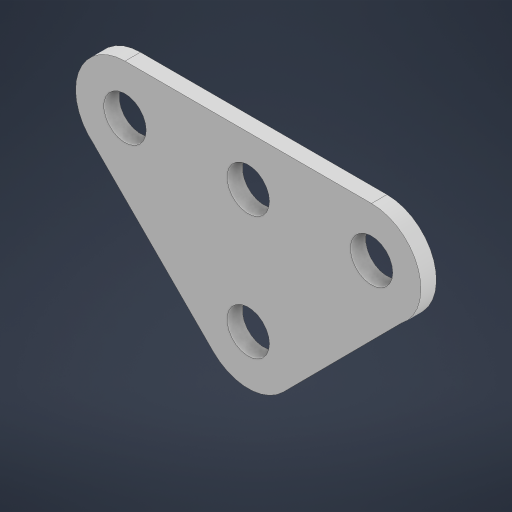
# Autodesk Inventor part: Wing poly connection
Saved by Autodesk Inventor 2023.4 (Build 274418000, 418)
## iProperties
Created: 2024-01-13
Part Number: Wing poly connection
Material: Generic
Document SubType Name: Modeling
Designer: diego
Density: 1 g/cm^3
Appearance: Default
Author: diego
Autodesk Inventor part; units mm, degrees
ref_plane "YZ Plane" through (0, 0, 0) normal (1, 0, 0) x (0, 1, 0)
ref_plane "XZ Plane" through (0, 0, 0) normal (0, 1, 0) x (-1, 0, 0)
ref_plane "XY Plane" through (0, 0, 0) normal (0, 0, 1) x (1, 0, 0)
sketch "Sketch1" plane through (0, 0, 0) normal (0, 0, 1) x (1, 0, 0)
  circle A0 centre (-20.2654, 5.4343) radius 2.1794
  line L0 (17.7594, 10.5431) -> (17.7594, 10.5431)
  line L1 (-10.775, 1.4678) -> (20.8786, 1.4678)
  line L2 (2.9338, -12.3151) -> (10.9845, -12.3151)
  line L3 (17.7594, 5.4646) -> (17.7594, 5.4646)
  circle A1 centre (17.7631, 5.4631) radius 5.08
  circle A2 centre (17.7631, 5.4631) radius 2.1844
  line L4 (17.7631, 5.4631) -> (5.0708, 5.4631)
  circle A3 centre (5.0708, 5.4631) radius 5.08
  circle A4 centre (5.0708, 5.4631) radius 2.1844
  line L5 (5.0708, 5.4631) -> (-7.6175, 5.4631)
  circle A5 centre (-7.6175, 5.4631) radius 5.08
  circle A6 centre (-7.6175, 5.4631) radius 2.1844
  line L6 (-7.6175, 10.5431) -> (5.0708, 10.5431)
  line L7 (5.0708, 10.5431) -> (17.7594, 10.5431)
  line L8 (5.0708, 5.4631) -> (5.0708, -7.2268)
  circle A7 centre (5.0708, -7.2268) radius 5.08
  circle A8 centre (5.0708, -7.2268) radius 2.1844
  line L9 (-10.775, 1.4678) -> (1.4683, -10.8085)
  line L10 (1.4683, -10.8085) -> (8.6733, -10.8085)
  line L11 (20.8786, 1.4678) -> (8.6733, -10.8085)
  point P0 (0, 0)
  point P1 (1.4353, -10.8085)
  point P2 (7.2024, -12.3151)
  point P3 (14.6256, 1.4678)
  point P4 (20.808, 1.3969)
  point P5 (-10.7549, 1.4678)
  dimension "d34" = 10.16
  dimension "d36" = 10.16
  dimension "d30" = 10.16
  dimension "d31" = 4.3688
  dimension "d35" = 4.3688
  dimension "d37" = 4.3688
  dimension "d38" = 10.16
  dimension "d39" = 4.3688
  constraints: 24 end point, 8 horizontal, 7 centre point, 7 coincident, 2 point on circle, 2 tangent, 1 point on line, 1 vertical, 1 vertical alignment, 5 other
  measures "d30" diameter of A1
  measures "d31" diameter of A2
  measures "d35" diameter of A4
  measures "d37" diameter of A6
  measures "d38" diameter of A7
  measures "d39" diameter of A8
extrude "Extrusion5" add sketch "Sketch1" along normal blind 1.5875 contours L1 A5 A3 L8 A7 L9 | A5 L1 | L1 A5 | L10 A7 | A7 L10 | A5 L5 A3 L1 | L6 A3 L5 A5 | A7 L8 A3 L1 A1 L11 | A3 L5 A4 L8 L1 | L1 L8 A3 | L7 A1 L4 A3 | A3 L4 A4 L5 | L11 L1 A1 | A1 L1 L11 | L8 L1 A3 | L8 A4 L4 A3 L1 | L4 A1 L1 A3
body "Solid5"
